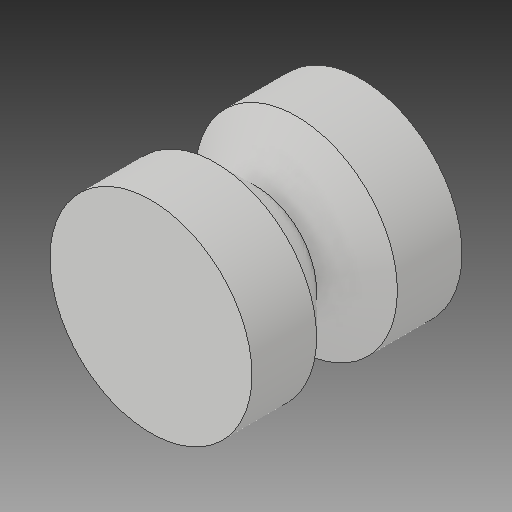
# Autodesk Inventor part: LiftPully
Saved by Autodesk Inventor 2019 (Build 230136000, 136)
## iProperties
Created: 2017-02-01
Part Number: LiftPully
Material: Generic
Document SubType Name: Modeling
Designer: RoboticsUser
Density: 1 g/cm^3
Appearance: Default
Mass: 1.45006 g
Surface Area: 8.06956 cm^2
Volume: 1.45006 cm^3
Author: RoboticsUser
Autodesk Inventor part; units mm, degrees
ref_plane "YZ Plane" through (0, 0, 0) normal (1, 0, 0) x (0, 1, 0)
ref_plane "XZ Plane" through (0, 0, 0) normal (0, 1, 0) x (-1, 0, 0)
ref_plane "XY Plane" through (0, 0, 0) normal (0, 0, 1) x (1, 0, 0)
sketch "Sketch1" plane through (0, 0, 0) normal (0, 0, 1) x (1, 0, 0)
  circle A0 centre (0, 0) radius 6.35
  dimension "d0" = 12.7
  constraints: 1 centre point, 1 coincident
  measures "d0" diameter of A0
extrude "Extrusion1" add sketch "Sketch1" along normal blind 6.604
chamfer "Chamfer1" distance 2.54 angle 45 1 edges at (-6.35, 0, 6.604)
sketch "Sketch2" plane through (0, 0, 6.604) normal (0, 0, 1) x (1, 0, 0)
  circle A0 centre (0, 0) radius 6.35
  dimension "d6" = 12.7
  constraints: 1 centre point, 1 coincident
  measures "d6" diameter of A0
extrude "Extrusion2" add sketch "Sketch2" along normal blind 6.604
chamfer "Chamfer2" distance 2.54 angle 45 1 edges at (-6.35, 0, 6.604)
body "Solid1"
